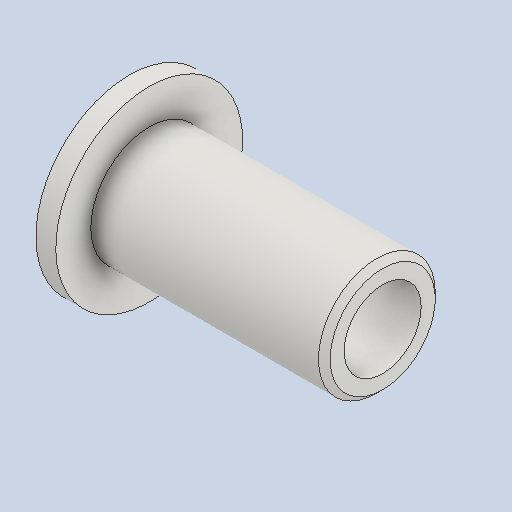
# Autodesk Inventor part: Wał
Saved by Autodesk Inventor 2023 (Build 270158000, 158)
## iProperties
CustomPartVersion: 1
Created: 2023-05-22
Part Number: Wał
Material: Steel
Document SubType Name: Modeling
Designer: krzys
Density: 1 g/cm^3
Appearance: Steel
Length: 21,700 mm
Author: krzys
Autodesk Inventor part; units mm, degrees
ref_plane "Płaszczyzna początkowa" through (0, 0, 0) normal (1, 0, 0) x (0, 1, 0)
ref_plane "XZ Plane" through (0, 0, 0) normal (0, 1, 0) x (-1, 0, 0)
ref_plane "XY Plane" through (0, 0, 0) normal (0, 0, 1) x (1, 0, 0)
sketch "Szkic główny" plane through (0, 0, 0) normal (0, 0, 1) x (1, 0, 0)
  line L0 (0, 0) -> (21.7, 0)
  line L1 (0, 0) -> (0, 8)
  line L2 (1.7, 8) -> (1.7, 5)
  line L3 (0, 8) -> (1.7, 8)
  line L4 (21.7, 5) -> (21.7, 0)
  line L5 (1.7, 5) -> (21.7, 5)
  dimension "d3" = 16
  dimension "d4" = 10
  constraints: 12 end point, 4 horizontal, 3 vertical
  measures "d3" diameter of L3 L0
  measures "d4" diameter of L5 L0
revolve "Obrót1" add sketch "Szkic główny" angle 360 about axis through (0, 0, 0) along (1, 0, 0)
chamfer "Faza1" distance 0.5 angle 45 1 edges at (21.7, -5, 0) measured on face at (15.0333, 4.9353, -0.8021)
sketch "Szkic3" plane through (21.7, 0, 0) normal (1, 0, 0) x (0, 0, -1)
  point P0 (0, 0)
hole "Otwór1" at (21.7, 0, 0) direction (-1, 0, 0) diameter 6.6 depth 21.7
sketch "Szkic4" plane through (21.7, 0, 0) normal (1, 0, 0) x (0, 0, -1)
  point P0 (0, 0)
hole "Otwór2" at (21.7, 0, 0) direction (-1, 0, 0) diameter 6.6 depth 21.7
equation "\"Length\" = 21.7"
